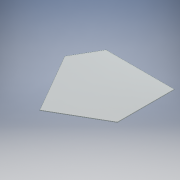
# Autodesk Inventor part: alu plate
Saved by Autodesk Inventor 2016 SP1 (Build 200210100, 210)
## iProperties
Created: 2016-04-14
Part Number: alu plate
Material: Glass
Document SubType Name: Modeling
Designer: ubik
Density: 2.18 g/cm^3
Appearance: Clear
Author: ubik
Autodesk Inventor part; units mm, degrees
ref_plane "YZ Plane" through (0, 0, 0) normal (1, 0, 0) x (0, 1, 0)
ref_plane "XZ Plane" through (0, 0, 0) normal (0, 1, 0) x (-1, 0, 0)
ref_plane "XY Plane" through (0, 0, 0) normal (0, 0, 1) x (1, 0, 0)
sketch "Sketch1" plane through (0, 0, 0) normal (0, 0, 1) x (1, 0, 0)
  arc A0 (-16.5011, 13.8506) -> (-21.6973, 4.8506) centre (-16.5011, 7.8506) ccw projected
  line L0 (-16.5011, 13.8506) -> (16.5011, 13.8506) projected
  arc A1 (21.6973, 4.8506) -> (16.5011, 13.8506) centre (16.5011, 7.8506) ccw projected
  line L1 (21.6973, 4.8506) -> (13.3257, -9.6494) projected
  arc A2 (5.5315, -14.1494) -> (13.3257, -9.6494) centre (5.5315, -5.1494) ccw projected
  line L2 (5.5315, -14.1494) -> (-5.5315, -14.1494) projected
  arc A3 (-13.3257, -9.6494) -> (-5.5315, -14.1494) centre (-5.5315, -5.1494) ccw projected
  line L3 (-13.3257, -9.6494) -> (-21.6973, 4.8506) projected
  line L4 (10, -20.5494) -> (10, -40.5494) projected
  line L5 (10, -40.5494) -> (-10, -40.5494) projected
  line L6 (-10, -40.5494) -> (-10, -20.5494) projected
  line L7 (-10, -20.5494) -> (10, -20.5494) projected
  line L8 (-43, 31.7481) -> (-15, -16.7494) projected
  line L9 (-15, -16.7494) -> (-32.2735, -26.7222) projected
  arc A4 (-32.2735, -26.7222) -> (32.2735, -26.7222) centre (0, -5.7301) ccw projected
  line L10 (32.2735, -26.7222) -> (15, -16.7494) projected
  line L11 (15, -16.7494) -> (43, 31.7481) projected
  line L12 (43, 31.7481) -> (38.6699, 34.2481) projected
  line L13 (38.6699, 34.2481) -> (31.7143, 22.2006) projected
  arc A5 (23.4871, 17.4506) -> (31.7143, 22.2006) centre (23.4871, 26.9506) ccw projected
  line L14 (23.4871, 17.4506) -> (-23.4871, 17.4506) projected
  arc A6 (-31.7143, 22.2006) -> (-23.4871, 17.4506) centre (-23.4871, 26.9506) ccw projected
  line L15 (-31.7143, 22.2006) -> (-38.6699, 34.2481) projected
  line L16 (-38.6699, 34.2481) -> (-43, 31.7481) projected
  arc A7 (-222.7491, 428.2441) -> (-227.9453, 437.2441) centre (-227.9453, 431.2441) ccw projected
  line L17 (-222.7491, 428.2441) -> (-239.2502, 399.6633) projected
  arc A8 (-249.6425, 399.6633) -> (-239.2502, 399.6633) centre (-244.4464, 402.6633) ccw projected
  line L18 (-249.6425, 399.6633) -> (-258.0141, 414.1633) projected
  arc A9 (-258.0141, 423.1633) -> (-258.0141, 414.1633) centre (-250.2199, 418.6633) ccw projected
  line L19 (-258.0141, 423.1633) -> (-252.4827, 432.7441) projected
  arc A10 (-244.6884, 437.2441) -> (-252.4827, 432.7441) centre (-244.6884, 428.2441) ccw projected
  line L20 (-244.6884, 437.2441) -> (-227.9453, 437.2441) projected
  line L21 (-265.791, 422.4934) -> (-283.1115, 432.4934) projected
  line L22 (-283.1115, 432.4934) -> (-273.1115, 449.8139) projected
  line L23 (-273.1115, 449.8139) -> (-255.791, 439.8139) projected
  line L24 (-255.791, 439.8139) -> (-265.791, 422.4934) projected
  line L25 (-194.0001, 442.2441) -> (-250.0001, 442.2441) projected
  line L26 (-250.0001, 442.2441) -> (-250.0001, 462.1898) projected
  arc A11 (-250.0001, 462.1898) -> (-282.2736, 406.2904) centre (-247.9571, 423.7441) ccw projected
  line L27 (-282.2736, 406.2904) -> (-265.0001, 416.2633) projected
  line L28 (-265.0001, 416.2633) -> (-237.0001, 367.7659) projected
  line L29 (-237.0001, 367.7659) -> (-232.6699, 370.2659) projected
  line L30 (-232.6699, 370.2659) -> (-239.6255, 382.3133) projected
  arc A12 (-239.6255, 391.8133) -> (-239.6255, 382.3133) centre (-231.3983, 387.0633) ccw projected
  line L31 (-239.6255, 391.8133) -> (-216.1385, 432.4941) projected
  arc A13 (-207.9112, 437.2441) -> (-216.1385, 432.4941) centre (-207.9112, 427.7441) ccw projected
  line L32 (-207.9112, 437.2441) -> (-194.0001, 437.2441) projected
  line L33 (-194.0001, 437.2441) -> (-194.0001, 442.2441) projected
  arc A14 (239.2501, 399.6635) -> (249.6424, 399.6635) centre (244.4463, 402.6635) ccw projected
  line L34 (239.2501, 399.6635) -> (222.749, 428.2443) projected
  arc A15 (227.9452, 437.2443) -> (222.749, 428.2443) centre (227.9452, 431.2443) ccw projected
  line L35 (227.9452, 437.2443) -> (244.6883, 437.2443) projected
  arc A16 (252.4825, 432.7443) -> (244.6883, 437.2443) centre (244.6883, 428.2443) ccw projected
  line L36 (252.4825, 432.7443) -> (258.014, 423.1635) projected
  arc A17 (258.014, 414.1635) -> (258.014, 423.1635) centre (250.2198, 418.6635) ccw projected
  line L37 (258.014, 414.1635) -> (249.6424, 399.6635) projected
  line L38 (255.7908, 439.8142) -> (273.1113, 449.8142) projected
  line L39 (273.1113, 449.8142) -> (283.1113, 432.4937) projected
  line L40 (283.1113, 432.4937) -> (265.7908, 422.4937) projected
  line L41 (265.7908, 422.4937) -> (255.7908, 439.8142) projected
  line L42 (237, 367.7661) -> (264.9999, 416.2635) projected
  line L43 (264.9999, 416.2635) -> (282.2735, 406.2907) projected
  arc A18 (282.2735, 406.2907) -> (249.9999, 462.19) centre (247.957, 423.7443) ccw projected
  line L44 (249.9999, 462.19) -> (249.9999, 442.2443) projected
  line L45 (249.9999, 442.2443) -> (193.9999, 442.2443) projected
  line L46 (193.9999, 442.2443) -> (193.9999, 437.2443) projected
  line L47 (193.9999, 437.2443) -> (207.9111, 437.2443) projected
  arc A19 (216.1383, 432.4943) -> (207.9111, 437.2443) centre (207.9111, 427.7443) ccw projected
  line L48 (216.1383, 432.4943) -> (239.6254, 391.8135) projected
  arc A20 (239.6254, 382.3135) -> (239.6254, 391.8135) centre (231.3982, 387.0635) ccw projected
  line L49 (239.6254, 382.3135) -> (232.6699, 370.2661) projected
  line L50 (232.6699, 370.2661) -> (237, 367.7661) projected
  line L51 (-194.0001, 442.2441) -> (193.9999, 442.2443)
  line L52 (193.9999, 442.2443) -> (237, 367.7661)
  line L53 (237, 367.7661) -> (43, 31.7481)
  line L54 (43, 31.7481) -> (-43, 31.7481)
  line L55 (-43, 31.7481) -> (-237.0001, 367.7659)
  line L56 (-237.0001, 367.7659) -> (-194.0001, 442.2441)
  line L57 (-247.9571, 423.7441) -> (0, 280.5861)
  line L58 (247.957, 423.7443) -> (0, 280.5861)
  line L59 (0, -5.7301) -> (0, 280.5861)
  line L60 (0, 280.5861) -> (140, 199.7571)
  line L61 (0, 280.5861) -> (-140, 199.757)
  line L62 (0, 280.5861) -> (-0.0001, 442.2442)
  point P0 (0, 0)
  constraints: 24 end point, 3 midpoint, 2 perpendicular, 1 collinear, 1 horizontal, 1 parallel
extrude "Extrusion1" add sketch "Sketch1" along normal blind 1.5 contours L61 L55 L29 L30 L56 L57 | L57 L56 L32 L33 L51 L62 | L30 L29 L56 | L56 L33 L32
body "Solid1"
